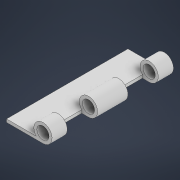
# Autodesk Inventor part: Poker hinge 1
Saved by Autodesk Inventor 2022 (Build 260153000, 153)
## iProperties
Created: 2021-05-25
Part Number: Poker hinge 1
Material: Generic
Document SubType Name: Modeling
Designer: Albert L Tomberg
Density: 1 g/cm^3
Appearance: Default
Author: Albert L Tomberg
Autodesk Inventor part; units mm, degrees
ref_plane "YZ Plane" through (0, 0, 0) normal (1, 0, 0) x (0, 1, 0)
sketch "Sketch1" plane through (0, 0, 0) normal (0, 0, 1) x (1, 0, 0)
  line L0 (0, 0) -> (-12, 0)
  line L1 (-12, 0) -> (-12, 1)
  line L2 (-12, 1) -> (-2.2361, 1)
  arc A0 (0, 0) -> (-2.2361, 1) centre (0, 3) ccw
  circle A1 centre (0, 3) radius 2
  dimension "d1" = 1
  dimension "d2" = 6
  dimension "d3" = 4
  dimension "d4" = 12
  constraints: 6 end point, 2 centre point, 2 point on circle, 1 coincident, 1 horizontal, 1 parallel, 1 perpendicular, 1 tangent
  measures "d1" distance of L0.end L1.end
  measures "d2" diameter of A0
  measures "d3" diameter of A1
  measures "d4" distance of L0.start L0.end
extrude "Extrusion1" add sketch "Sketch1" against normal blind 40
ref_plane "Work Plane1" through (0, 0, -5) normal (0, 0, 1) x (1, 0, 0)
sketch "Sketch3" plane through (0, 0, -5) normal (0, 0, 1) x (1, 0, 0)
  arc A0 (0, 0) -> (-2.2361, 1) centre (0, 3) ccw projected
  arc A1 (0, 0) -> (-2.2361, 1) centre (0, 3) ccw projected
  line L0 (-2.2361, 1) -> (-2.2361, 0)
  line L1 (-2.2361, 0) -> (0, 0)
  circle A2 centre (0, 3) radius 2 projected
  circle A3 centre (0, 3) radius 2 projected
  point P0 (-2.2361, 1)
  constraints: 4 end point, 1 perpendicular, 1 vertical
extrude "Extrusion2" cut sketch "Sketch3" against normal blind 10
ref_plane "Work Plane2" through (0, 0, -35) normal (0, 0, -1) x (-1, 0, 0)
sketch "Sketch4" plane through (0, 0, -35) normal (0, 0, -1) x (-1, 0, 0)
  arc A0 (2.2361, 1) -> (0, 0) centre (0, 3) ccw projected
  arc A1 (2.2361, 1) -> (0, 0) centre (0, 3) ccw projected
  circle A2 centre (0, 3) radius 2 projected
  circle A3 centre (0, 3) radius 2 projected
  line L0 (2.2361, 1) -> (2.2361, 0)
  line L1 (2.2361, 0) -> (0, 0)
  point P0 (2.2361, 1)
  constraints: 4 end point, 1 perpendicular, 1 vertical
extrude "Extrusion3" cut sketch "Sketch4" against normal blind 10
body "Solid1"
